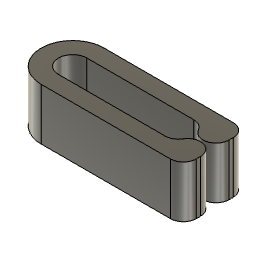
cable holder (Autodesk Fusion 360 design; units mm, degrees)
Autodesk Fusion 360 part; units mm, degrees
sketch "Sketch1" plane through (0, 0, 0) normal (0, 0, 1) x (1, 0, 0)
  circle A0 centre (0, 0) radius 1.65
  circle A1 centre (0, 0) radius 3.65
  line L0 (0, 0) -> (0, -3.65)
  line L1 (0, 0) -> (0, 3.65)
  line L2 (0, 3.65) -> (15, 3.65)
  line L3 (0, -3.65) -> (15, -3.65)
  line L4 (0, 1.65) -> (12.4019, 1.65)
  line L5 (0, -1.65) -> (12.4019, -1.65)
  line L6 (16.5, 2.15) -> (16.5, 1.65)
  line L7 (16.5, -2.15) -> (16.5, -1.65)
  arc A2 (15, -0.15) -> (13.701, -0.9) centre (15, -1.65) ccw
  arc A3 (16.5, -1.65) -> (15, -0.15) centre (15, -1.65) ccw
  arc A4 (13.701, 0.9) -> (15, 0.15) centre (15, 1.65) ccw
  arc A5 (15, 0.15) -> (16.5, 1.65) centre (15, 1.65) ccw
  arc A6 (13.701, 0.9) -> (12.4019, 1.65) centre (12.4019, 0.15) ccw
  arc A7 (12.4019, -1.65) -> (13.701, -0.9) centre (12.4019, -0.15) ccw
  arc A8 (15, -3.65) -> (16.5, -2.15) centre (15, -2.15) ccw
  arc A9 (16.5, 2.15) -> (15, 3.65) centre (15, 2.15) ccw
  point P0 (16.5, 3.65)
  point P1 (16.5, -3.65)
  point P2 (13.5, 1.65)
  point P3 (13.5, -1.65)
  point P4 (16.5, 3.65)
  point P5 (16.5, 0.15)
  point P6 (16.5, -3.65)
  point P7 (16.5, -0.15)
  point P8 (13.5, 0.15)
  point P9 (13.5, -0.15)
  dimension "d1" = 3.3
  dimension "d2" = 7.3
  dimension "d10" = 16.5
  dimension "d11" = 16.5
  dimension "d18" = 13.5
  dimension "d19" = 13.5
  dimension "d23" = 3.5
  dimension "d24" = 3.5
  dimension "d25" = 3
  dimension "d26" = 3
  dimension "d27" = 1.5
  dimension "d28" = 1.5
  dimension "d29" = 1.5
  dimension "d30" = 1.5
  dimension "d31" = 1.5
  dimension "d32" = 1.5
  dimension "d33" = 1.5
  dimension "d34" = 1.5
  constraint coincident A0.centre A1.centre
  constraint concentric A0 A1
  constraint coincident A1 L0.end
  constraint vertical L0
  constraint coincident A1 L1.end
  constraint parallel L0 L1
  constraint perpendicular L1 L2
  constraint perpendicular L0 L3
  constraint coincident P4 L2
  constraint coincident P6 L3
  constraint coincident L1 L4.start
  constraint coincident A0 L4.start
  constraint perpendicular L1 L4
  constraint coincident A0 L5.start
  constraint coincident L0 L5.start
  constraint perpendicular L0 L5
  constraint coincident P4 P0
  constraint perpendicular L2 L6
  constraint coincident P6 P1
  constraint perpendicular L3 L7
  constraint coincident P7 L7
  constraint tangent L7 A3
  constraint coincident A2.start A3.end
  constraint coincident P5 L6
  constraint tangent L6 A5
  constraint coincident A4.end A5.start
  constraint tangent A4 A6
  constraint tangent L4 A6
  constraint tangent L5 A7
  constraint tangent A2 A7
  constraint coincident P6 L7
  constraint tangent L3 A8
  constraint tangent L7 A8
  constraint coincident P4 L6
  constraint tangent L2 A9
  constraint tangent L6 A9
  measures "d1" diameter of A0
  measures "d2" diameter of A1
  measures "d10" distance of L1.end P4
  measures "d11" distance of L0.end P6
  measures "d18" distance of L4.start P2
  measures "d19" distance of L5.start P3
  measures "d23" distance of P4 P5
  measures "d24" distance of P6 P7
  measures "d25" distance of P5 P8
  measures "d26" distance of P7 P9
  measures "d27" radius of A2
  measures "d28" radius of A3
  measures "d29" radius of A4
  measures "d30" radius of A5
  measures "d31" radius of A6
  measures "d32" radius of A7
  measures "d33" radius of A8
  measures "d34" radius of A9
extrude "Extrude4" add sketch "Sketch1" along normal blind 6 contours A0 A1 L0 L1 | A1 L1 L4 | A1 L0 L5 | A1 L2 L4 L6 A4 A5 A6 A9 | A1 L3 L5 L7 A2 A3 A7 A8
